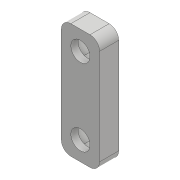
# Autodesk Inventor part: connector_brace
Saved by Autodesk Inventor 2017 (Build 210142000, 142)
## iProperties
Created: 2018-07-01
Part Number: connector_brace
Material: Generic
Document SubType Name: Modeling
Designer: mfans
Density: 1 g/cm^3
Appearance: Default
Author: mfans
Autodesk Inventor part; units mm, degrees
ref_plane "YZ Plane" through (0, 0, 0) normal (1, 0, 0) x (0, 1, 0)
ref_plane "XZ Plane" through (0, 0, 0) normal (0, 1, 0) x (-1, 0, 0)
ref_plane "XY Plane" through (0, 0, 0) normal (0, 0, 1) x (1, 0, 0)
sketch "Sketch1" plane through (0, 0, 0) normal (0, 1, 0) x (-1, 0, 0)
  line L0 (-4, 12) -> (4, 12)
  line L1 (4, 12) -> (4, -12)
  line L2 (4, -12) -> (-4, -12)
  line L3 (-4, -12) -> (-4, 12)
  line L4 (-4, 12) -> (4, -12) construction
  line L5 (4, 12) -> (-4, -12) construction
  point P0 (0, 0)
  dimension "d0" = 8
  dimension "d1" = 24
  constraints: 12 end point, 2 midpoint, 2 parallel, 1 horizontal, 1 perpendicular
  measures "d0" distance of L1.end L2.end
  measures "d1" distance of L0.end L1.end
extrude "Extrusion1" add sketch "Sketch1" along normal blind 4
sketch "Sketch2" plane through (0, 4, 0) normal (0, 1, 0) x (1, 0, 0)
  line L0 (3.1754, -8) -> (1.5877, -10.75)
  line L1 (1.5877, -10.75) -> (-1.5877, -10.75)
  line L2 (-1.5877, -10.75) -> (-3.1754, -8)
  line L3 (-3.1754, -8) -> (-1.5877, -5.25)
  line L4 (-1.5877, -5.25) -> (1.5877, -5.25)
  line L5 (1.5877, -5.25) -> (3.1754, -8)
  line L6 (-4, -12) -> (4, -12) projected
  line L7 (-4, 12) -> (-4, -12) projected
  line L8 (-4, 0) -> (4, 0)
  line L9 (3.1754, 8) -> (1.5877, 10.75)
  line L10 (1.5877, 10.75) -> (-1.5877, 10.75)
  line L11 (-1.5877, 10.75) -> (-3.1754, 8)
  line L12 (-3.1754, 8) -> (-1.5877, 5.25)
  line L13 (-1.5877, 5.25) -> (1.5877, 5.25)
  line L14 (1.5877, 5.25) -> (3.1754, 8)
  point P0 (0, 0)
  point P1 (0, -8)
  dimension "d4" = 0
  dimension "d5" = 8
  dimension "d6" = 5.5
  constraints: 26 end point, 6 symmetric about line, 1 horizontal, 1 midpoint, 1 parallel, 13 other
  measures "d4" horizontal distance of point (0, 0) point (0, -8)
  measures "d5" distance of point (0, 0) point (0, -8)
  measures "d6" distance between parallel lines of L1 L4
extrude "Extrusion2" cut sketch "Sketch2" against normal blind 2.5
fillet "Fillet1" radius 2 4 edges at (4, 2, 12) (-4, 2, 12) (4, 2, -12) (-4, 2, -12)
sketch "Sketch3" plane through (0, 1.5, 0) normal (0, 1, 0) x (1, 0, 0)
  line L0 (3.1754, -8) -> (1.5877, -10.75) projected
  line L1 (1.5877, -5.25) -> (3.1754, -8) projected
  line L2 (-1.5877, -5.25) -> (1.5877, -5.25) projected
  line L3 (-3.1754, -8) -> (-1.5877, -5.25) projected
  line L4 (-1.5877, -10.75) -> (-3.1754, -8) projected
  line L5 (1.5877, -10.75) -> (-1.5877, -10.75) projected
  line L6 (-3.1754, 8) -> (-1.5877, 10.75) projected
  line L7 (-1.5877, 5.25) -> (-3.1754, 8) projected
  line L8 (1.5877, 5.25) -> (-1.5877, 5.25) projected
  line L9 (3.1754, 8) -> (1.5877, 5.25) projected
  line L10 (1.5877, 10.75) -> (3.1754, 8) projected
  line L11 (-1.5877, 10.75) -> (1.5877, 10.75) projected
  point P0 (0, 0)
  point P1 (0, -8)
  point P2 (0, 8)
hole "Hole1" at (0, 1.5, 8) at (0, 1.5, -8) direction (0, -1, 0) diameter 4 end through all
body "Solid1"
